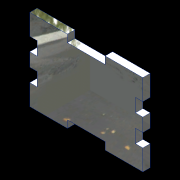
# Autodesk Inventor part: FrontDriveArmorPlate
Saved by Autodesk Inventor 2022 (Build 260153000, 153)
## iProperties
Created: 2022-03-07
Part Number: FrontDriveArmorPlate
Material: Aluminum 6061
Document SubType Name: Modeling
Designer: tandu
Density: 2.7 g/cm^3
Appearance: Aluminum - Flat
Author: tandu
Autodesk Inventor part; units mm, degrees
ref_plane "YZ Plane" through (0, 0, 0) normal (1, 0, 0) x (0, 1, 0)
ref_plane "XZ Plane" through (0, 0, 0) normal (0, 1, 0) x (-1, 0, 0)
ref_plane "Work Plane1" through (0, 0, 0) normal (0, 0, 1) x (1, 0, 0)
sketch "Sketch1" plane through (0, 0, 0) normal (0, 0, 1) x (1, 0, 0)
  line L0 (19.05, 25.4) -> (-149.225, 25.4) construction
  line L1 (19.1104, -88.9) -> (-149.1646, -88.9) construction
  line L2 (-149.225, 25.4) -> (19.1104, 25.4) construction
  line L3 (19.1104, 25.4) -> (19.1104, -88.9) construction
  line L4 (19.1104, -88.9) -> (-149.225, -88.9) construction
  line L5 (-149.225, -88.9) -> (-149.225, 25.4) construction
  line L6 (19.05, 25.4) -> (31.75, 25.4) projected
  line L7 (31.75, 25.4) -> (31.75, 2.54) projected
  line L8 (19.05, 2.54) -> (31.75, 2.54) projected
  line L9 (19.05, 2.54) -> (19.05, -20.32) projected
  line L10 (19.05, -20.32) -> (31.75, -20.32) projected
  line L11 (31.75, -20.32) -> (31.75, -43.18) projected
  line L12 (19.05, -43.18) -> (31.75, -43.18) projected
  line L13 (19.05, -43.18) -> (19.05, -66.04) projected
  line L14 (31.75, -66.04) -> (31.75, -88.9) projected
  line L15 (19.05, -88.9) -> (31.75, -88.9) projected
  line L16 (-65.0573, 25.4) -> (-65.0573, -88.9) construction
  line L17 (31.75, -31.75) -> (-149.225, -31.75) construction
  line L18 (19.05, -66.04) -> (31.75, -66.04) projected
  line L19 (-149.1646, 25.4) -> (-161.8646, 25.4)
  line L20 (-161.8646, 25.4) -> (-161.8646, 2.54)
  line L21 (-149.1646, 2.54) -> (-161.8646, 2.54)
  line L22 (-149.1646, 2.54) -> (-149.1646, -20.32)
  line L23 (-149.1646, -20.32) -> (-161.8646, -20.32)
  line L24 (-161.8646, -20.32) -> (-161.8646, -43.18)
  line L25 (-149.1646, -43.18) -> (-161.8646, -43.18)
  line L26 (-149.1646, -43.18) -> (-149.1646, -66.04)
  line L27 (-161.8646, -66.04) -> (-161.8646, -88.9)
  line L28 (-149.1646, -88.9) -> (-161.8646, -88.9)
  line L29 (-149.1646, -66.04) -> (-161.8646, -66.04)
  line L30 (31.75, 25.4) -> (19.1104, 25.4) construction
  line L31 (31.75, -88.9) -> (19.05, -88.9) construction
  line L32 (-161.8646, 25.4) -> (-97.3264, 25.4) construction
  line L33 (-97.3264, 25.4) -> (-97.3264, 38.1)
  line L34 (-97.3264, 38.1) -> (-161.8646, 38.1)
  line L35 (-161.8646, 38.1) -> (-161.8646, 25.4)
  line L36 (-97.3264, 25.4) -> (-32.7882, 25.4)
  line L37 (-32.7882, 25.4) -> (-32.7882, 38.1)
  line L38 (-32.7882, 38.1) -> (-97.3264, 38.1)
  line L39 (-97.3264, 38.1) -> (-97.3264, 25.4)
  line L40 (-32.7882, 25.4) -> (31.75, 25.4) construction
  line L41 (31.75, 25.4) -> (31.75, 38.1)
  line L42 (31.75, 38.1) -> (-32.7882, 38.1)
  line L43 (-32.7882, 38.1) -> (-32.7882, 25.4)
  line L44 (-97.3264, -101.6) -> (-161.8646, -101.6)
  line L45 (-161.8646, -101.6) -> (-161.8646, -88.9)
  line L46 (-97.3264, -88.9) -> (-32.7882, -88.9)
  line L47 (-97.3264, -101.6) -> (-97.3264, -88.9)
  line L48 (31.75, -88.9) -> (31.75, -101.6)
  line L49 (31.75, -101.6) -> (-32.7882, -101.6)
  line L50 (-32.7882, -88.9) -> (-32.7882, -101.6)
  point P0 (0, 0)
  dimension "d0" = 12.7
  constraints: 76 end point, 19 symmetric about line, 8 parallel, 4 collinear, 4 horizontal, 4 midpoint, 4 perpendicular, 2 point on line
  measures "d0" distance of L6.end L41.end
extrude "Extrusion1" add sketch "Sketch1" along normal blind 12.7 contours L7 L8 L9 L10 L11 L12 L13 L18 L14 L48 L49 L50 L46 L47 L44 L45 L27 L29 L26 L25 L24 L23 L22 L21 L20 L35 L34 L33 L36 L37 L42 L41
equation "\"d1\" = Thickness"
equation "\"Thickness\" = 12.7"
body "Solid1"
